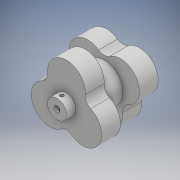
# Autodesk Inventor part: field-mover
Saved by Autodesk Inventor 2017 (Build 210142000, 142)
## iProperties
Created: 2017-03-05
Part Number: field-mover
Material: Generic
Document SubType Name: Modeling
Designer: John
Density: 1 g/cm^3
Appearance: Default
Author: John
Autodesk Inventor part; units mm, degrees
ref_plane "YZ Plane" through (0, 0, 0) normal (1, 0, 0) x (0, 1, 0)
ref_plane "XZ Plane" through (0, 0, 0) normal (0, 1, 0) x (-1, 0, 0)
ref_plane "XY Plane" through (0, 0, 0) normal (0, 0, 1) x (1, 0, 0)
sketch "Sketch1" plane through (0, 0, 0) normal (0, 1, 0) x (-1, 0, 0)
  circle A0 centre (0, 0) radius 20 construction
  circle A1 centre (0, 20) radius 20
  circle A2 centre (0, 0) radius 20 construction
  circle A3 centre (-17.3205, -10) radius 20
  circle A4 centre (0, 0) radius 20 construction
  circle A5 centre (17.3205, -10) radius 20
  dimension "d0" = 40
  dimension "d1" = 40
  dimension "d4" = 360
  constraints: 5 coincident, 3 centre point, 1 vertical alignment, 22 other
  measures "d1" diameter of A1
extrude "Extrusion1" add sketch "Sketch1" along normal blind 20
fillet "Fillet1" radius 10 1 edges at (0, 10, -20)
fillet "Fillet2" radius 10 1 edges at (-17.3205, 10, 10)
fillet "Fillet3" radius 10 1 edges at (17.3205, 10, 10)
sketch "Sketch2" plane through (0, 0, 0) normal (0, 1, 0) x (-1, 0, 0)
  circle A0 centre (0, 0) radius 10
  dimension "d11" = 20
  constraints: 1 centre point, 1 coincident
  measures "d11" diameter of A0
extrude "Extrusion2" add sketch "Sketch2" against normal blind 10
sketch "Sketch3" plane through (0, 0, 0) normal (0, 0, 1) x (1, 0, 0)
  circle A0 centre (0, -5) radius 2
  line L0 (-10, -10) -> (10, -10) projected
  point P0 (0, 0)
  dimension "d14" = 4
  dimension "d15" = 5
  constraints: 1 centre point
  measures "d14" diameter of A0
  measures "d15" distance from line of L0 A0.centre
extrude "Extrusion3" cut sketch "Sketch3" along normal through all both and the other way through all
sketch "Sketch4" plane through (0, -10, 0) normal (0, -1, 0) x (1, 0, 0)
  circle A0 centre (0, 0) radius 3.25
  dimension "d18" = 6.5
  constraints: 1 centre point, 1 coincident
  measures "d18" diameter of A0
extrude "Extrusion4" cut sketch "Sketch4" against normal blind 15
sketch "Sketch6" plane through (0, 20, 0) normal (0, 1, 0) x (1, 0, 0)
  circle A0 centre (0, 0) radius 20
  dimension "d26" = 40
  constraints: 1 centre point, 1 coincident
  measures "d26" diameter of A0
extrude "Extrusion5" add sketch "Sketch6" along normal blind 20
sketch "Sketch7" plane through (0, 40, 0) normal (0, 1, 0) x (1, 0, 0)
  circle A0 centre (0, 0) radius 20 construction
  circle A1 centre (0, 20) radius 20
  circle A2 centre (0, 0) radius 20 construction
  circle A3 centre (-17.3205, -10) radius 20
  circle A4 centre (0, 0) radius 20 construction
  circle A5 centre (17.3205, -10) radius 20
  dimension "d31" = 40
  dimension "d32" = 40
  dimension "d33" = 360
  constraints: 5 coincident, 3 centre point, 1 vertical alignment, 22 other
  measures "d32" diameter of A1
extrude "Extrusion6" add sketch "Sketch7" along normal blind 20
fillet "Fillet4" radius 10 3 edges at (17.3205, 50, -10) (-17.3205, 50, -10) (0, 50, 20)
equation "\"d1\" = d0"
equation "\"d32\" = d31"
body "Solid1"
